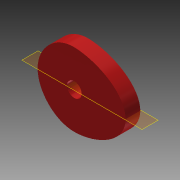
# Autodesk Inventor part: Cam lobe
Saved by Autodesk Inventor 2015 (Build 190141000, 141)
## iProperties
Created: 2008-06-10
Part Number: Cam lobe
Document SubType Name: Modeling
Designer: tangg
Density: 7.75 g/cm^3
Mass: 5.71787 g
Surface Area: 26.2129 cm^2
Volume: 5.71787 cm^3
Stock Number: Cam lobe
Material: Stainless Steel, 440C
Appearance: Light Red
Author: tangg
Autodesk Inventor part; units mm, degrees
ref_plane "YZ Plane" through (0, 0, 0) normal (1, 0, 0) x (0, 1, 0)
ref_plane "XY Plane" through (0, 0, 0) normal (0, 0, 1) x (1, 0, 0)
sketch "Sketch1" plane through (0, 0, 0) normal (0, 0, 1) x (1, 0, 0)
  circle A0 centre (0, 0) radius 3.175
  line L0 (-0.0081, 11.43) -> (-0.0081, -11.43) construction
  line L1 (-0.0081, 0.0081) -> (15.875, -15.875) construction
  line L2 (0, 0) -> (13.5171, 13.5171) construction
  spline S0 degree 4 poles (0, 15.875) (-4.7386, 16.0053) (-12.159, 12.4629) (-20.0222, 0.064) (-12.1399, -12.4984) (-4.7192, -15.875) (0, -15.875) knots 0 0 0 0 0 0.374971 0.624971 1 1 1 1 1
  line L3 (-0.0081, 0.0081) -> (-14.3755, 14.3755) construction
  line L4 (0, 0) -> (-13.1389, -13.1389) construction
  spline S1 degree 4 poles (0, 15.875) (7.4077, 15.6714) (27.0977, 8.786) (27.2968, -8.7181) (7.2086, -15.875) (0, -15.875) knots 0 0 0 0 0 0.5 1 1 1 1 1
  line L5 (22.225, 3.8294) -> (22.225, -3.8294) construction
  arc A1 (21.7894, -2.9312) -> (21.7894, 2.9312) centre (12.1443, 0) ccw construction
  line L6 (4.981, -15.875) -> (-4.981, -15.875) construction
  arc A2 (-3.903, -15.4775) -> (3.903, -15.4775) centre (0, 3.487) ccw construction
  point P0 (-0.0081, 0)
  point P1 (-11.1125, 11.1125)
  point P2 (-15.869, 0.0264)
  point P3 (-11.0968, -11.0727)
  point P4 (22.225, 0)
  dimension "d0" = 6.35
  dimension "d7" = 45
  dimension "d8" = 45
  dimension "d9" = 45
  dimension "d10" = 45
  constraints: 14 end point, 5 midpoint, 3 centre point, 3 point on line, 3 vertical, 2 horizontal, 2 point on circle, 1 coincident, 12 other
  measures "d0" diameter of A0
  measures "d7" angle of L0 L1
  measures "d8" angle of L0 L2
  measures "d9" angle of L4 L0
  measures "d10" angle of L3 L0
extrude "Extrusion1" add sketch "Sketch1" along normal blind 6.35
sketch "Sketch4" plane through (0, 0, 0) normal (0, 1, 0) x (-1, 0, 0)
  point P0 (0, 0)
sketch "Sketch5" plane through (0, 0, 0) normal (0, 1, 0) x (-1, 0, 0)
  point P0 (0, 0)
body "Solid1"
